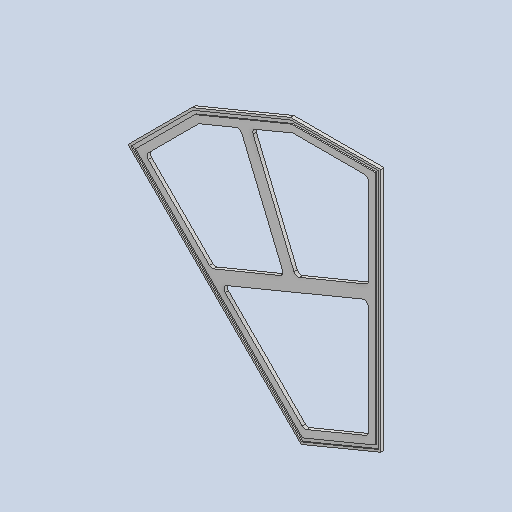
# Autodesk Inventor part: ДМФ 0121 Внешняя рамка
Saved by Autodesk Inventor 2024.2 (Build 282272000, 272)
## iProperties
Created: 2024-05-05
Part Number: ДМФ 0121 Внешняя рамка
Material: Generic
Document SubType Name: Modeling
Designer: pokla
Density: 1 g/cm^3
Appearance: Default
Author: pokla
Autodesk Inventor part; units mm, degrees
ref_plane "YZ Plane" through (0, 0, 0) normal (1, 0, 0) x (0, 1, 0)
ref_plane "XZ Plane" through (0, 0, 0) normal (0, 1, 0) x (-1, 0, 0)
ref_plane "XY Plane" through (0, 0, 0) normal (0, 0, 1) x (1, 0, 0)
sketch "Sketch1" plane through (0, 0, 0) normal (0, 0, 1) x (1, 0, 0)
  line L0 (0, 273.8452) -> (193.6378, 193.6378) construction
  line L1 (193.6378, 193.6378) -> (273.8452, 0) construction
  line L2 (273.8452, 0) -> (193.6378, -193.6378) construction
  line L3 (193.6378, -193.6378) -> (0, -273.8452) construction
  line L4 (0, -273.8452) -> (-193.6378, -193.6378) construction
  line L5 (-193.6378, -193.6378) -> (-273.8452, 0) construction
  line L6 (-273.8452, 0) -> (-193.6378, 193.6378) construction
  line L7 (-193.6378, 193.6378) -> (0, 273.8452)
  line L8 (-193.6378, 193.6378) -> (0, 273.8452)
  line L9 (-459.9272, 770.6562) -> (-219.7185, 870.1539)
  line L10 (-96.8189, 233.7415) -> (-339.8229, 820.405) construction
  line L11 (-219.7185, 870.1539) -> (0, 870.1539)
  line L12 (0, 870.1539) -> (0, 273.8452)
  line L13 (-459.9272, 770.6562) -> (-615.2917, 615.2917)
  line L14 (-615.2917, 615.2917) -> (-193.6378, 193.6378)
  point P0 (0, 0)
  point P1 (0, 0)
  dimension "d0" = 506
  dimension "d2" = 260
  dimension "d3" = 635
  constraints: 30 end point, 2 midpoint, 1 coincident, 1 horizontal, 1 parallel, 1 perpendicular, 1 symmetric about line, 1 vertical, 1 vertical alignment, 17 other
  measures "d0" distance between parallel lines of L5 L1
  measures "d2" distance of L9.start L9.end
  measures "d3" distance of L10.end L10.start
extrude "Extrusion1" add sketch "Sketch1" along normal mid plane 8
sketch "Sketch2" plane through (0, 0, 4) normal (0, 0, 1) x (1, 0, 0)
  line L0 (-219.7185, 870.1539) -> (-459.9272, 770.6562) projected
  line L1 (-459.9272, 770.6562) -> (-615.2917, 615.2917) projected
  line L2 (-235.0492, 528.2621) -> (-412.382, 454.8085)
  line L3 (-193.6378, 193.6378) -> (0, 273.8452) projected
  line L4 (-96.8189, 233.7415) -> (-339.8229, 820.405) construction
  line L5 (-615.2917, 615.2917) -> (-193.6378, 193.6378) projected
  line L6 (-412.382, 454.8085) -> (-572.8653, 615.2917)
  line L7 (-572.8653, 615.2917) -> (-442.9336, 745.2234)
  line L8 (-442.9336, 745.2234) -> (-342.2006, 786.9484)
  line L9 (-235.0492, 528.2621) -> (-342.2006, 786.9484)
  line L10 (-207.3328, 539.7426) -> (-30, 613.1963)
  line L11 (-30, 613.1963) -> (-30, 840.1539)
  line L12 (-30, 840.1539) -> (-213.7512, 840.1539)
  line L13 (-213.7512, 840.1539) -> (-314.4842, 798.4289)
  line L14 (-207.3328, 539.7426) -> (-314.4842, 798.4289)
  line L15 (0, 273.8452) -> (0, 870.1539) projected
  line L16 (-412.382, 454.8085) -> (-30, 613.1963) construction
  line L17 (-389.421, 431.8474) -> (-30, 580.7245)
  line L18 (-186.5988, 229.0252) -> (-30, 293.8906)
  line L19 (-30, 293.8906) -> (-30, 580.7245)
  line L20 (-186.5988, 229.0252) -> (-389.421, 431.8474)
  point P0 (0, 0)
  dimension "d11" = 30
  dimension "d12" = 280
  dimension "d13" = 30
  dimension "d14" = 30
  dimension "d15" = 15
  dimension "d21" = 30
  dimension "d22" = 30
  dimension "d23" = 30
  dimension "d24" = 30
  constraints: 32 end point, 5 parallel, 5 symmetric about line, 2 midpoint, 1 collinear
  measures "d11" distance between parallel lines of L5 L6
  measures "d12" distance between parallel lines of L8 L2
  measures "d13" distance between parallel lines of L0 L8
  measures "d14" distance between parallel lines of L1 L7
  measures "d15" distance between parallel lines of L9 L4
  measures "d21" distance between parallel lines of L16 L17
  measures "d22" distance between parallel lines of L5 L20
  measures "d23" distance between parallel lines of L19 L15
  measures "d24" distance between parallel lines of L18 L3
extrude "Extrusion2" cut sketch "Sketch2" against normal up to surface (8 mm away)
fillet "Fillet1" radius 10 12 edges at (-572.8653, 615.2917, 0) (-342.2006, 786.9484, 0) (-235.0492, 528.2621, 0) (-412.382, 454.8085, 0) (-314.4842, 798.4289, 0) (-30, 840.1539, 0) (-30, 613.1963, 0) (-207.3328, 539.7426, 0) (-389.421, 431.8474, 0) (-30, 580.7245, 0) (-30, 293.8906, 0) (-186.5988, 229.0252, 0)
sketch "Sketch4" plane through (0, 0, 4) normal (0, 0, 1) x (1, 0, 0)
  line L0 (-219.7185, 870.1539) -> (-459.9272, 770.6562) projected
  line L1 (0, 870.1539) -> (-219.7185, 870.1539) projected
  line L2 (-459.9272, 770.6562) -> (-615.2917, 615.2917) projected
  line L3 (-615.2917, 615.2917) -> (-193.6378, 193.6378) projected
  line L4 (-193.6378, 193.6378) -> (0, 273.8452) projected
  line L5 (0, 273.8452) -> (0, 870.1539) projected
  line L6 (-457.095, 766.4174) -> (-218.724, 865.1539)
  line L7 (-218.724, 865.1539) -> (-5, 865.1539)
  line L8 (-5, 865.1539) -> (-5, 277.1861)
  line L9 (-5, 277.1861) -> (-192.4647, 199.5357)
  line L10 (-192.4647, 199.5357) -> (-608.2206, 615.2917)
  line L11 (-608.2206, 615.2917) -> (-457.095, 766.4174)
  line L12 (-217.1327, 857.1539) -> (-452.5633, 759.6353)
  line L13 (-452.5633, 759.6353) -> (-596.9069, 615.2917)
  line L14 (-596.9069, 615.2917) -> (-190.5876, 208.9724)
  line L15 (-190.5876, 208.9724) -> (-13, 282.5315)
  line L16 (-13, 282.5315) -> (-13, 857.1539)
  line L17 (-13, 857.1539) -> (-217.1327, 857.1539)
  point P0 (0, 0)
  dimension "d26" = 5
  dimension "d27" = 8
  constraints: 24 end point, 10 other
  measures "d26" distance between parallel lines of L0 L6
  measures "d27" distance between parallel lines of L6 L12
extrude "Extrusion3" cut sketch "Sketch4" against normal blind 3 contours L6 L7 L8 L9 L10 L11
fillet "Fillet3" radius 16 2 edges at (-218.724, 865.1539, 2.5) (-457.095, 766.4174, 2.5)
fillet "Fillet4" radius 8 2 edges at (-452.5633, 759.6353, 2.5) (-217.1327, 857.1539, 2.5)
equation "\"d0\" = Барабан_габарит_по_кассетам"
equation "\"d2\" = Кассета_длина_грани"
equation "\"d3\" = Кассета_высота"
equation "\"d11\" = d13"
equation "\"d14\" = d13"
equation "\"d15\" = 0.5 * d13"
equation "\"d21\" = d13"
equation "\"d22\" = d13"
equation "\"d23\" = d13"
equation "\"d24\" = d13"
equation "\"Барабан_габарит_по_кассетам\" = 506"
equation "\"Кассета_длина_грани\" = 260"
equation "\"Кассета_высота\" = 635"
body "Solid1"
